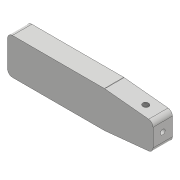
# Autodesk Inventor part: Switch_Extend
Saved by Autodesk Inventor 2018 (Build 220112000, 112)
## iProperties
Created: 2019-11-23
Part Number: Switch_Extend
Material: Generic
Document SubType Name: Modeling
Designer: Clevo
Density: 1 g/cm^3
Appearance: Default
Author: Clevo
Autodesk Inventor part; units mm, degrees
ref_plane "YZ Plane" through (0, 0, 0) normal (1, 0, 0) x (0, 1, 0)
ref_plane "XZ Plane" through (0, 0, 0) normal (0, 1, 0) x (-1, 0, 0)
ref_plane "XY Plane" through (0, 0, 0) normal (0, 0, 1) x (1, 0, 0)
sketch "Sketch1" plane through (0, 0, 0) normal (0, 1, 0) x (-1, 0, 0)
  line L0 (-30, -7.5) -> (30, -7.5)
  line L1 (30, -7.5) -> (30, 7.5)
  line L2 (30, 7.5) -> (-30, 7.5)
  line L3 (-30, 7.5) -> (-30, -7.5)
  line L4 (-30, -7.5) -> (30, 7.5) construction
  line L5 (30, -7.5) -> (-30, 7.5) construction
  point P0 (0, 0)
  dimension "d0" = 15
  dimension "d1" = 60
  constraints: 12 end point, 2 midpoint, 2 parallel, 1 horizontal, 1 perpendicular
  measures "d0" distance of L0.end L1.end
  measures "d1" distance of L1.end L2.end
extrude "Extrusion1" add sketch "Sketch1" along normal mid plane 8
sketch "Sketch2" plane through (0, 4, 0) normal (0, 1, 0) x (1, 0, 0)
  line L0 (30, 7.5) -> (-30, 7.5) projected
  line L1 (-30, 7.5) -> (-30, -7.5) projected
  line L2 (-30, -7.5) -> (30, -7.5) projected
  line L3 (30, -7.5) -> (30, 7.5) projected
  line L4 (-30, -7.5) -> (30, -7.5) projected
  line L5 (10, -7.5) -> (30, -5.5)
  line L6 (30, -7.5) -> (30, 7.5) projected
  point P0 (0, 0)
  dimension "d4" = 20
  dimension "d5" = 2
  constraints: 2 end point, 2 point on line
  measures "d4" distance from line of L3 L5.start
  measures "d5" distance from line of L2 L5.end
extrude "Extrusion2" cut sketch "Sketch2" against normal through all contours L3 L2 L5
mirror "Mirror1" about plane through (0, 0, 0) normal (0, 0, 1) of "Extrusion2"
fillet "Fillet1" radius 2 6 edges at (-30, 0, 7.5) (-30, 0, -7.5) (10, 0, -7.5) (10, 0, 7.5) (30, 0, 5.5) (30, 0, -5.5)
sketch "Sketch3" plane through (30, -4, 3.69) normal (1, 0, 0) x (0, 0, -1)
  line L0 (7.38, 8) -> (7.38, 0) projected
  line L1 (0, 8) -> (7.38, 8) projected
  line L2 (0, 0) -> (0, 8) projected
  line L3 (7.38, 0) -> (0, 0) projected
  line L4 (7.38, 8) -> (0, 8)
  line L5 (0, 8) -> (0, 0)
  line L6 (0, 0) -> (7.38, 0)
  line L7 (7.38, 0) -> (7.38, 8)
  line L8 (7.38, 8) -> (0, 0) construction
  line L9 (0, 8) -> (7.38, 0) construction
  point P0 (3.69, 4)
  point P1 (3.69, 4)
  constraints: 12 end point, 2 midpoint, 2 parallel, 1 horizontal, 1 perpendicular
hole "Hole1" at (30, 0, 0) direction (-1, 0, 0) diameter 2 depth 8 tip angle 118
sketch "Sketch4" plane through (-28, -4, 7.5) normal (0, 0, 1) x (1, 0, 0)
  line L0 (58, 0) -> (58, 8) projected
  point P0 (28, 4)
  point P1 (51, 4)
  point P2 (58, 4)
  dimension "d16" = 7
  constraints: 1 horizontal alignment, 1 midpoint
  measures "d16" distance from line of L0 point (51, 4)
hole "Hole2" at (23, 0, 7.5) direction (0, 0, -1) diameter 2.459 end through all thread size "M3x0.5" class "6H" standard "ANSI Metric M Profile"
body "Solid1"
